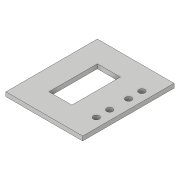
# Autodesk Inventor part: switch holder
Saved by Autodesk Inventor 2018 (Build 220112000, 112)
## iProperties
Created: 2017-12-14
Part Number: switch holder
Material: Generic
Document SubType Name: Modeling
Designer: ball
Density: 1 g/cm^3
Appearance: Default
Author: ball
Autodesk Inventor part; units mm, degrees
ref_plane "YZ Plane" through (0, 0, 0) normal (1, 0, 0) x (0, 1, 0)
ref_plane "XZ Plane" through (0, 0, 0) normal (0, 1, 0) x (-1, 0, 0)
ref_plane "XY Plane" through (0, 0, 0) normal (0, 0, 1) x (1, 0, 0)
sketch "Sketch1" plane through (0, 0, 0) normal (0, 1, 0) x (-1, 0, 0)
  line L0 (-22.6949, -27.051) -> (22.6949, -27.051)
  line L1 (22.6949, -27.051) -> (22.6949, 27.051)
  line L2 (22.6949, 27.051) -> (-22.6949, 27.051)
  line L3 (-22.6949, 27.051) -> (-22.6949, -27.051)
  line L4 (-22.6949, -27.051) -> (22.6949, 27.051) construction
  line L5 (22.6949, -27.051) -> (-22.6949, 27.051) construction
  point P0 (0, 0)
  dimension "d0" = 45.3898
  dimension "d1" = 54.102
  constraints: 12 end point, 2 midpoint, 2 parallel, 1 horizontal, 1 perpendicular
  measures "d0" distance between parallel lines of L1 L3
  measures "d1" distance between parallel lines of L0 L2
extrude "Extrusion1" add sketch "Sketch1" along normal blind 2.54
sketch "Sketch2" plane through (0, 2.54, 0) normal (0, 1, 0) x (1, 0, 0)
  line L0 (-9.9949, 14.351) -> (3.6449, 14.351)
  line L1 (3.6449, 14.351) -> (3.6449, -14.351)
  line L2 (3.6449, -14.351) -> (-9.9949, -14.351)
  line L3 (-9.9949, -14.351) -> (-9.9949, 14.351)
  line L4 (22.6949, -27.051) -> (22.6949, 27.051) projected
  line L5 (22.6949, 27.051) -> (-22.6949, 27.051) projected
  point P0 (0, 0)
  dimension "d4" = 13.6398
  dimension "d5" = 28.702
  dimension "d6" = 19.05
  dimension "d7" = 12.7
  constraints: 8 end point, 2 parallel, 1 horizontal, 1 perpendicular
  measures "d4" distance of L0.start L0.end
  measures "d5" distance of L2.end L0.start
  measures "d6" distance between parallel lines of L4 L1
  measures "d7" distance between parallel lines of L5 L0
extrude "Extrusion2" cut sketch "Sketch2" against normal through all
sketch "Sketch3" plane through (0, 2.54, 0) normal (0, 1, 0) x (1, 0, 0)
  circle A0 centre (17.2339, -5.588) radius 1.778
  line L0 (22.6949, -27.051) -> (22.6949, 27.051) projected
  circle A1 centre (17.2339, 5.588) radius 1.778
  circle A2 centre (17.2339, 13.4747) radius 1.778
  circle A3 centre (17.2339, -13.4747) radius 1.778
  line L1 (-22.6949, -27.051) -> (22.6949, -27.051) projected
  line L2 (22.6949, 27.051) -> (-22.6949, 27.051) projected
  point P0 (0, 0)
  dimension "d10" = 3.556
  dimension "d12" = 3.556
  dimension "d13" = 14.732
  dimension "d14" = 7.62
  dimension "d15" = 3.556
  dimension "d16" = 3.556
  dimension "d17" = 4.3307
  dimension "d18" = 4.3307
  dimension "d19" = 26.9494
  dimension "d20" = 13.5763
  dimension "d21" = 13.5763
  constraints: 4 centre point
  measures "d10" diameter of A0
  measures "d12" diameter of A1
  measures "d15" diameter of A2
  measures "d16" diameter of A3
  measures "d19" distance of A2.centre A3.centre
  measures "d20" distance from line of L1 A3.centre
  measures "d21" distance from line of L2 A2.centre
extrude "Extrusion3" cut sketch "Sketch3" against normal through all
body "Solid1"
